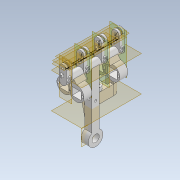
# Autodesk Inventor part: base_hand
Saved by Autodesk Inventor 2020.2 (Build 242310000, 310)
## iProperties
Created: 2020-04-08
Part Number: base_hand
Material: Generic
Document SubType Name: Modeling
Designer: Bardo91
Density: 1 g/cm^3
Appearance: Default
Author: Bardo91
Autodesk Inventor part; units mm, degrees
ref_plane "YZ Plane" through (0, 0, 0) normal (1, 0, 0) x (0, 1, 0)
sketch "Sketch1" plane through (0, 0, 0) normal (1, 0, 0) x (0, 1, 0)
  line L0 (0, 0) -> (0, -24)
  line L1 (0, -24) -> (0, -48)
  line L2 (0, -48) -> (0, -72)
  line L3 (0, -24) -> (5, -24)
  line L4 (0, -48) -> (8, -48)
  line L5 (0, -72) -> (5, -72)
  dimension "d0" = 24
  dimension "d1" = 24
  dimension "d2" = 24
  dimension "d4" = 5
  dimension "d5" = 8
  dimension "d6" = 5
  constraints: 12 end point, 2 horizontal, 2 point on line, 1 perpendicular, 1 vertical
  measures "d0" distance of L0.start L0.end
  measures "d1" distance of L0.end L1.end
  measures "d2" distance of L1.end L2.end
  measures "d4" distance of L0.end L3.end
  measures "d5" distance of L1.end L4.end
  measures "d6" distance of L2.end L5.end
ref_plane "Work Plane1" through (0, 5, -24) normal (0, 0, 1) x (1, 0, 0)
ref_plane "Work Plane3" through (0, 5, -72) normal (0, 0, 1) x (1, 0, 0)
ref_plane "Work Plane2" through (0, 8, -48) normal (0, 0, 1) x (1, 0, 0)
ref_plane "Work Plane4" through (0, 0, 0) normal (0, 0, 1) x (1, 0, 0)
sketch "Sketch2" plane through (0, 0, 0) normal (0, 0, 1) x (1, 0, 0)
  circle A0 centre (0, 0) radius 1.5
  circle A1 centre (0, 0) radius 5
  line L0 (0, 0) -> (0, -15)
  circle A2 centre (0, -15) radius 5
  line L1 (5, -15) -> (5, 0)
  line L2 (-5, -15) -> (-5, 0)
  dimension "d7" = 3
  dimension "d8" = 10
  dimension "d80" = 15
  dimension "d81" = 10
  constraints: 6 end point, 4 point on circle, 3 centre point, 3 coincident, 2 tangent, 2 vertical, 1 parallel
  measures "d7" diameter of A0
  measures "d8" diameter of A1
  measures "d80" distance of L0.start L0.end
  measures "d81" diameter of A2
extrude "pinky_joint" add sketch "Sketch2" along normal mid plane 8
sketch "Sketch18" plane through (0, 0, 4) normal (0, 0, 1) x (1, 0, 0)
  line L0 (0, 0) -> (0, -6)
  line L1 (0, -6) -> (0, -9)
  line L2 (0, 0) -> (1.058, -6)
  line L3 (0, 0) -> (6.0926, 0) construction
  line L4 (1.058, -6) -> (0, -6)
  line L5 (1.058, -6) -> (1.5869, -9)
  line L6 (1.5869, -9) -> (0, -9)
  dimension "d82" = 6
  dimension "d83" = 3
  dimension "d84" = 80
  constraints: 14 end point, 2 horizontal, 2 point on line, 1 equal length, 1 parallel, 1 vertical
  measures "d82" distance of L0.start L0.end
  measures "d83" distance of L0.end L1.end
  measures "d84" angle of L2 L3
extrude "lock" add sketch "Sketch18" along normal blind 3 contours L4 L5 L6 L1
ref_plane "Work Plane5" through (0, 0, 0) normal (0, 0, 1) x (1, 0, 0)
mirror "Mirror1" about plane through (0, 0, 0) normal (0, 0, 1) of "lock"
chamfer "Chamfer1" distance 3 angle 45 2 edges at (0, -7.5, 4) (0, -7.5, -4)
ref_plane "Work Plane6" through (0, 5, 0) normal (0, 1, 0) x (-1, 0, 0)
sketch "Sketch19" plane through (0, 5, 0) normal (0, 1, 0) x (-1, 0, 0)
  line L0 (0, 0) -> (-3, 0)
  circle A0 centre (-3, 0) radius 1.25
  dimension "d90" = 3
  dimension "thread_hole" = 2.5
  constraints: 2 end point, 1 centre point, 1 coincident, 1 horizontal
  measures "d90" distance of L0.start L0.end
  measures "thread_hole" diameter of A0
extrude "thread_hole" cut sketch "Sketch19" against normal through all
sketch "Sketch20" plane through (0, 0, 0) normal (0, 1, 0) x (-1, 0, 0)
  line L0 (0, 0) -> (-3, 0)
  circle A0 centre (-3, 0) radius 1.25
  line L1 (-3, -1.25) -> (-5, -1.25)
  line L2 (-5, -4) -> (-5, 4) projected
  line L3 (-3, 1.25) -> (-5, 1.25)
  line L4 (0, 0) -> (0, 2.405)
  dimension "d94" = 3
  dimension "d95" = 2.5
  constraints: 8 end point, 2 horizontal, 2 point on circle, 2 point on line, 1 centre point, 1 coincident, 1 parallel, 1 vertical
  measures "d94" distance of L0.start L0.end
  measures "d95" diameter of A0
revolve "Revolution2" cut sketch "Sketch20" angle 180 about axis through (0, 0, 0) along (0, 0, 1)
sketch "Sketch22" plane through (5, -15, 4) normal (1, 0, 0) x (0, 0, -1)
  line L0 (8, 0) -> (0, 0) projected
  line L1 (4, 0) -> (4, 1)
  circle A0 centre (4, 1) radius 1
  line L2 (4, 1) -> (4, 5)
  circle A1 centre (4, 5) radius 1
  point P0 (4, 15)
  dimension "d100" = 1
  dimension "d101" = 2
  dimension "d104" = 4
  dimension "d105" = 2
  constraints: 4 end point, 2 centre point, 2 coincident, 2 vertical, 1 midpoint
  measures "d100" distance of L1.start L1.end
  measures "d101" diameter of A0
  measures "d104" distance of L2.start L2.end
  measures "d105" diameter of A1
extrude "pinky_flector_holder" cut sketch "Sketch22" against normal up to surface round surface about axis through (3, 5, 0) along (0, -1, 0) radius 1.25 far side no
sketch "Sketch23" plane through (0, 0, -4) normal (0, 0, -1) x (-1, 0, 0)
  arc A0 (-5, -15) -> (5, -15) centre (0, -15) ccw projected
  circle A1 centre (0, -15) radius 5
  point P0 (0, 0)
  constraints: 1 coincident, 3 other
extrude "finger_union" add sketch "Sketch23" along normal blind 72
sketch "Sketch24" plane through (-5, 0, -1.25) normal (0, 1, 0) x (1, 0, 0)
  arc A0 (2, -2.5) -> (2, 0) centre (2, -1.25) ccw projected
  circle A1 centre (2, -1.25) radius 1.25
  point P0 (5, -1.25)
  constraints: 1 coincident, 3 other
extrude "pinky_actuator_hole" cut sketch "Sketch24" against normal through all
ref_plane "Work Plane7" through (0, 5, -24) normal (0, 0, -1) x (-1, 0, 0)
sketch "Sketch25" plane through (0, 5, -24) normal (0, 0, -1) x (-1, 0, 0)
  arc A0 (5, -5) -> (-5, -5) centre (0, -5) ccw projected
  circle A1 centre (0, 0) radius 1.5
  circle A2 centre (0, 0) radius 5
  line L0 (5, -5) -> (5, -20) projected
  line L1 (5, 0) -> (5, -20)
  line L2 (-5, -20) -> (-5, -5) projected
  line L3 (-5, 0) -> (-5, -20)
  circle A3 centre (0, -20) radius 5 projected
  circle A4 centre (0, -20) radius 5
  point P0 (-5, -5)
  point P1 (5, -5)
  dimension "d112" = 3
  dimension "d113" = 10
  constraints: 4 end point, 3 point on circle, 2 centre point, 2 coincident, 2 collinear, 1 horizontal alignment, 2 other
  measures "d112" diameter of A1
  measures "d113" diameter of A2
extrude "ring_base" add sketch "Sketch25" along normal mid plane 8 contours L0 A3 L2 A0 A2 | A0 A2 L1 | A2 A0 A1 | A0 A1 A2 | A0 L3 A2
sketch "Sketch26" plane through (0, 5, -20) normal (0, 0, 1) x (1, 0, 0)
  line L0 (0, 0) -> (0, -6)
  line L1 (0, -6) -> (0, -9)
  line L2 (0, 0) -> (1.5869, -9)
  line L3 (0, 0) -> (9.1388, 0) construction
  line L4 (1.5869, -9) -> (0, -9)
  line L5 (0, -6) -> (1.058, -6)
  point P0 (0, -5)
  dimension "d116" = 6
  dimension "d117" = 3
  dimension "d118" = 80
  constraints: 12 end point, 2 horizontal, 2 vertical, 1 equal length, 1 parallel, 1 point on line
  measures "d116" distance of L0.start L0.end
  measures "d117" distance of L0.end L1.end
  measures "d118" angle of L2 L3
extrude "ring_lock" add sketch "Sketch26" along normal blind 3 contours L5 L2 L4 L1
mirror "Mirror2" about plane through (0, 5, -24) normal (0, 0, -1) of "ring_lock"
chamfer "Chamfer2" distance 3 angle 45 2 edges at (0, -2.5, -20) (0, -2.5, -28)
ref_plane "Work Plane8" through (0, 8, -48) normal (0, 0, -1) x (-1, 0, 0)
ref_plane "Work Plane9" through (0, 5, -72) normal (0, 0, -1) x (-1, 0, 0)
sketch "Sketch27" plane through (0, 8, -48) normal (0, 0, -1) x (-1, 0, 0)
  circle A0 centre (0, 0) radius 1.5
  circle A1 centre (0, 0) radius 5
  line L0 (5, -8) -> (5, -23) projected
  line L1 (5, 0) -> (5, -23)
  arc A2 (5, -23) -> (-5, -23) centre (0, -23) ccw projected
  line L2 (-5, 0) -> (-5, -23)
  point P0 (0, -8)
  point P1 (5, -8)
  dimension "d124" = 3
  dimension "d125" = 10
  constraints: 4 end point, 2 centre point, 2 point on circle, 2 vertical, 1 coincident, 1 tangent
  measures "d124" diameter of A0
  measures "d125" diameter of A1
extrude "middle_base" add sketch "Sketch27" along normal mid plane 8
ref_plane "Work Plane11" through (5, 8, -44) normal (0, 1, 0) x (-1, 0, 0)
ref_plane "Work Plane10" through (5, 5, -20) normal (0, 1, 0) x (-1, 0, 0)
sketch "Sketch28" plane through (0, 5, -72) normal (0, 0, -1) x (-1, 0, 0)
  circle A0 centre (0, 0) radius 1.5
  circle A1 centre (0, 0) radius 5
  line L0 (5, 3) -> (5, -20) projected
  line L1 (5, 0) -> (5, -20)
  line L2 (-5, -20) -> (-5, 3) projected
  line L3 (-5, 0) -> (-5, -20)
  arc A2 (5, -20) -> (-5, -20) centre (0, -20) ccw projected
  circle A3 centre (0, -20) radius 5
  point P0 (0, -5)
  dimension "d128" = 3
  dimension "d129" = 10
  constraints: 4 end point, 2 centre point, 2 coincident, 2 collinear, 2 point on circle, 2 point on line, 1 horizontal alignment, 1 tangent, 2 other
  measures "d128" diameter of A0
  measures "d129" diameter of A1
extrude "index_base" add sketch "Sketch28" along normal mid plane 8 contours A1 | L0 A2 L2 A1
sketch "Sketch39" plane through (5, 5, -20) normal (0, 1, 0) x (-1, 0, 0)
  line L0 (10, -8) -> (10, 0) projected
  line L1 (10, -4) -> (0, -4)
  line L2 (0, -8) -> (0, 0) projected
  line L3 (5, -4) -> (1.5, -4)
  circle A0 centre (1.5, -4) radius 1.25
  line L4 (1.5, -5.25) -> (0, -5.25)
  line L5 (1.5, -2.75) -> (0, -2.75)
  line L6 (5, -4) -> (5, -5.6429)
  line L7 (0, -5.25) -> (0, -2.75)
  point P0 (5, 20)
  dimension "d165" = 3.5
  dimension "d166" = 2.5
  constraints: 12 end point, 3 midpoint, 3 point on line, 2 perpendicular, 2 point on circle, 1 centre point, 1 coincident, 1 collinear, 1 tangent, 1 vertical
  measures "d165" distance of L3.start L3.end
  measures "d166" diameter of A0
revolve "ring_1" cut sketch "Sketch39" angle 180 about axis through (0, 5, -24) along (0, 0, 1)
sketch "Sketch40" plane through (3.5, 5, -22.75) normal (0, 1, 0) x (1, 0, 0)
  arc A0 (0, 2.5) -> (0, 0) centre (0, 1.25) ccw projected
  circle A1 centre (0, 1.25) radius 1.25
  point P0 (-3.5, -22.75)
  constraints: 1 coincident, 3 other
extrude "ring_2" cut sketch "Sketch40" against normal through all
sketch "Sketch41" plane through (5, -15, -28) normal (1, 0, 0) x (0, 0, -1)
  line L0 (0, 0) -> (-8, 0) projected
  line L1 (-4, 0) -> (-4, 1)
  line L2 (-4, 1) -> (-4, 5)
  circle A0 centre (-4, 5) radius 1
  circle A1 centre (-4, 1) radius 1
  point P0 (-28, 15)
  dimension "d170" = 1
  dimension "d171" = 4
  dimension "d172" = 2
  dimension "d173" = 2
  constraints: 4 end point, 2 centre point, 2 coincident, 1 midpoint, 1 point on line, 1 vertical
  measures "d170" distance of L1.start L1.end
  measures "d171" distance of L1.end L2.end
  measures "d172" diameter of A0
  measures "d173" diameter of A1
extrude "ring_3" cut sketch "Sketch41" against normal up to surface round surface about axis through (3.5, 5, -24) along (0, -1, 0) radius 1.25 far side no
sketch "Sketch42" plane through (-5, 5, -22.75) normal (0, 1, 0) x (1, 0, 0)
  arc A0 (1.5, 0) -> (1.5, 2.5) centre (1.5, 1.25) ccw projected
  circle A1 centre (1.5, 1.25) radius 1.25
  point P0 (5, -22.75)
  constraints: 1 coincident, 3 other
extrude "ring_4" cut sketch "Sketch42" against normal through all
sketch "Sketch30" plane through (5, 8, -44) normal (0, 1, 0) x (-1, 0, 0)
  line L0 (10, -8) -> (10, 0) projected
  line L1 (10, -4) -> (0, -4)
  line L2 (0, 0) -> (0, -8) projected
  line L3 (5, -4) -> (1.5, -4)
  circle A0 centre (1.5, -4) radius 1.25
  line L4 (1.5, -5.25) -> (0, -5.25)
  line L5 (1.5, -2.75) -> (0, -2.75)
  line L6 (5, -4) -> (5, -4.8662)
  point P0 (5, 44)
  dimension "d135" = 3.5
  dimension "d136" = 2.5
  constraints: 10 end point, 3 midpoint, 3 point on line, 2 point on circle, 1 centre point, 1 coincident, 1 parallel, 1 perpendicular, 1 tangent, 1 vertical
  measures "d135" distance of L3.start L3.end
  measures "d136" diameter of A0
revolve "middle_1" cut sketch "Sketch30" angle 180 about axis through (0, 8, -48) along (0, 0, 1)
sketch "Sketch34" plane through (3.5, 8, -49.25) normal (0, 1, 0) x (1, 0, 0)
  arc A0 (0, 0) -> (0, -2.5) centre (0, -1.25) ccw projected
  circle A1 centre (0, -1.25) radius 1.25
  point P0 (-3.5, -49.25)
  point P1 (0, -2.5)
  constraints: 1 coincident, 3 other
extrude "middle_2" cut sketch "Sketch34" against normal through all
sketch "Sketch35" plane through (5, -15, -52) normal (1, 0, 0) x (0, 0, -1)
  line L0 (0, 0) -> (-8, 0) projected
  line L1 (-4, 0) -> (-4, 1)
  line L2 (-4, 1) -> (-4, 5)
  circle A0 centre (-4, 1) radius 1
  circle A1 centre (-4, 5) radius 1
  point P0 (-52, 15)
  dimension "d151" = 1
  dimension "d152" = 4
  dimension "d153" = 2
  dimension "d154" = 2
  constraints: 4 end point, 2 centre point, 2 coincident, 1 midpoint, 1 point on line, 1 vertical
  measures "d151" distance of L1.start L1.end
  measures "d152" distance of L1.end L2.end
  measures "d153" diameter of A0
  measures "d154" diameter of A1
extrude "middle_3" cut sketch "Sketch35" against normal up to surface round surface about axis through (3.5, 8, -48) along (0, -1, 0) radius 1.25 far side no
sketch "Sketch43" plane through (-5, 8, -49.25) normal (0, 1, 0) x (1, 0, 0)
  arc A0 (1.5, -2.5) -> (1.5, 0) centre (1.5, -1.25) ccw projected
  circle A1 centre (1.5, -1.25) radius 1.25
  point P0 (5, -49.25)
  point P1 (1.5, 0)
  constraints: 1 centre point, 1 coincident
extrude "middle_4" cut sketch "Sketch43" against normal through all
sketch "Sketch31" plane through (5, 5, -20) normal (0, 1, 0) x (-1, 0, 0)
  line L0 (10, -48) -> (10, -56) projected
  line L1 (10, -52) -> (0, -52)
  line L2 (0, -56) -> (0, -48) projected
  line L3 (5, -52) -> (1.5, -52)
  circle A0 centre (1.5, -52) radius 1.25
  line L4 (1.5, -53.25) -> (0, -53.25)
  line L5 (1.5, -50.75) -> (0, -50.75)
  line L6 (5, -52) -> (5, -50.2742)
  point P0 (5, 20)
  dimension "d138" = 3.5
  dimension "d139" = 2.5
  constraints: 10 end point, 3 midpoint, 3 point on line, 2 perpendicular, 2 point on circle, 1 centre point, 1 coincident, 1 tangent, 1 vertical
  measures "d138" distance of L3.start L3.end
  measures "d139" diameter of A0
revolve "index_1" cut sketch "Sketch31" angle 180 about axis through (0, 5, -72) along (0, 0, 1)
sketch "Sketch36" plane through (3.5, 5, -70.75) normal (0, 1, 0) x (1, 0, 0)
  arc A0 (0, 2.5) -> (0, 0) centre (0, 1.25) ccw projected
  circle A1 centre (0, 1.25) radius 1.25
  point P0 (-3.5, -70.75)
  constraints: 1 coincident, 3 other
extrude "index_2" cut sketch "Sketch36" against normal through all
sketch "Sketch37" plane through (5, -15, -76) normal (1, 0, 0) x (0, 0, -1)
  line L0 (-4, 0) -> (-4, 1)
  line L1 (-4, 1) -> (-4, 5)
  circle A0 centre (-4, 5) radius 1
  circle A1 centre (-4, 1) radius 1
  line L2 (-8, 0) -> (-8, 20) projected
  line L3 (0, 0) -> (0, 20) projected
  point P0 (-76, 15)
  dimension "d159" = 1
  dimension "d160" = 4
  dimension "d161" = 2
  dimension "d162" = 2
  dimension "d434" = 4
  constraints: 4 end point, 2 centre point, 2 coincident, 1 point on line, 1 vertical
  measures "d159" distance of L0.start L0.end
  measures "d160" distance of L0.end L1.end
  measures "d161" diameter of A0
  measures "d162" diameter of A1
  measures "d434" distance between parallel lines of L3 L1
extrude "index_3" cut sketch "Sketch37" against normal up to surface round surface about axis through (3.5, 5, -72) along (0, -1, 0) radius 1.25 far side no
sketch "Sketch44" plane through (-5, 5, -70.75) normal (0, 1, 0) x (1, 0, 0)
  arc A0 (1.5, 0) -> (1.5, 2.5) centre (1.5, 1.25) ccw projected
  circle A1 centre (1.5, 1.25) radius 1.25
  point P0 (5, -70.75)
  point P1 (1.5, 0)
  constraints: 1 coincident, 3 other
extrude "index_4" cut sketch "Sketch44" against normal through all
sketch "Sketch46" plane through (0, 5, -20) normal (0, 0, 1) x (1, 0, 0)
  arc A0 (-5, -20) -> (5, -20) centre (0, -20) ccw projected
  circle A1 centre (9, -35) radius 10
  line L0 (9, -25) -> (5, -20)
  line L1 (-1, -35) -> (-5, -20)
  line L2 (9, -35) -> (15, -35)
  line L3 (15, -35) -> (15, -30)
  line L4 (15, -30) -> (3, -30)
  line L5 (3, -30) -> (3, -40)
  line L6 (3, -40) -> (15, -40)
  line L7 (15, -40) -> (15, -35)
  line L8 (15.2, -35) -> (15.2, -29.8)
  line L9 (15.2, -29.8) -> (2.8, -29.8)
  line L10 (2.8, -29.8) -> (2.8, -40.2)
  line L11 (2.8, -40.2) -> (15.2, -40.2)
  line L12 (15.2, -40.2) -> (15.2, -35)
  point P0 (0, -5)
  point P1 (18.9875, -34.5)
  point P2 (18.9875, -35.5)
  point P3 (-4.3361, -22.4896)
  dimension "d369" = 15
  dimension "d370" = 9
  dimension "d371" = 6
  dimension "d372" = 5
  dimension "d373" = 12
  dimension "d374" = 10
  dimension "d375" = 0.2
  constraints: 26 end point, 7 perpendicular, 5 point on circle, 2 collinear, 1 centre point, 1 horizontal, 1 point on line, 4 other
  measures "d369" vertical distance of A0.centre L2.start
  measures "d370" horizontal distance of A0.centre L2.start
  measures "d371" distance of L2.start L2.end
  measures "d372" distance of L2.end L3.end
  measures "d373" distance of L3.end L4.end
  measures "d374" distance of L4.end L5.end
  measures "d375" distance between parallel lines of L7 L12
sketch "Sketch51" plane through (0, 8, -52) normal (0, 0, -1) x (-1, 0, 0)
  arc A0 (-4.9962, -22.8052) -> (-4.9944, -22.7631) centre (0, -23) ccw
  line L0 (0, -23) -> (0, -38)
  line L1 (0, -38) -> (-9, -38)
  circle A1 centre (-9, -38) radius 10
  arc A2 (-5, -23) -> (5, -23) centre (0, -23) ccw projected
  line L2 (-9, -28) -> (-5, -23)
  line L3 (1, -38) -> (5, -23)
  line L4 (-9, -38) -> (-15, -38)
  line L5 (-15, -38) -> (-15, -33)
  line L6 (-15, -33) -> (-3, -33)
  line L7 (-3, -33) -> (-3, -43)
  line L8 (-3, -43) -> (-15, -43)
  line L9 (-15, -43) -> (-15, -38)
  line L10 (-2.8, -43.2) -> (-2.8, -32.8)
  line L11 (-2.8, -32.8) -> (-15.2, -32.8)
  line L12 (-15.2, -32.8) -> (-15.2, -38)
  line L13 (-15.2, -38) -> (-15.2, -43.2)
  line L14 (-15.2, -43.2) -> (-2.8, -43.2)
  point P0 (0, -5)
  point P1 (0, -5)
  point P2 (0.9875, -37.5)
  point P3 (-7.2605, -28.1524)
  point P4 (-5, -23)
  point P5 (5, -23)
  point P6 (4.3361, -25.4896)
  point P7 (-18.9875, -38.5)
  point P8 (-18.9875, -37.5)
  dimension "d227" = 15
  dimension "d230" = 20
  dimension "d235" = 5
  dimension "d237" = 9
  dimension "d382" = 6
  dimension "d383" = 5
  dimension "d384" = 12
  dimension "d385" = 10
  dimension "d386" = 0.2
  constraints: 30 end point, 10 perpendicular, 8 point on circle, 2 centre point, 2 coincident, 1 horizontal, 1 point on line, 1 vertical, 4 other
  measures "d227" distance of L0.start L0.end
  measures "d230" diameter of A1
  measures "d235" radius of A0
  measures "d237" distance of L0.end L1.end
  measures "d382" distance of L4.start L4.end
  measures "d383" distance of L4.end L5.end
  measures "d384" distance of L5.end L6.end
  measures "d385" distance of L6.end L7.end
  measures "d386" distance between parallel lines of L7 L10
extrude "ring_motor" add sketch "Sketch46" along normal blind 14 contours A0 L0 A1 L1 | A1
extrude "middle_motor" add sketch "Sketch51" along normal blind 14 contours A0 L0 A1 L2 | A0 L3 A1 L0 | A1
sketch "Sketch52" plane through (0, 5, -68) normal (0, 0, 1) x (1, 0, 0)
  arc A0 (-4.9995, -20.0687) -> (4.9995, -20.0687) centre (0, -20) ccw
  line L0 (0, -20) -> (0, -35)
  circle A1 centre (-9, -35) radius 10
  arc A2 (-4.3361, -22.4896) -> (5, -20) centre (0, -20) ccw projected
  line L1 (5, -20) -> (9, -25) projected
  line L2 (1, -35) -> (5, -20)
  line L3 (-4.3361, -22.4896) -> (-8.7782, -25.0025)
  line L4 (-9, -35) -> (-3, -35)
  line L5 (-3, -35) -> (-3, -40)
  line L6 (-3, -40) -> (-15, -40)
  line L7 (-15, -40) -> (-15, -30)
  line L8 (-15, -30) -> (-3, -30)
  line L9 (-3, -30) -> (-3, -35)
  line L10 (-2.8, -40.2) -> (-2.8, -35)
  line L11 (-2.8, -35) -> (-2.8, -29.8)
  line L12 (-2.8, -29.8) -> (-15.2, -29.8)
  line L13 (-15.2, -29.8) -> (-15.2, -40.2)
  line L14 (-15.2, -40.2) -> (-2.8, -40.2)
  point P0 (0, -5)
  point P1 (0, -5)
  point P2 (0.9875, -34.5)
  point P3 (0.9875, -35.5)
  point P4 (11.9791, -34.5)
  point P5 (11.9791, -35.5)
  point P6 (-4.9558, -20.6637)
  point P7 (4.3361, -22.4896)
  point P8 (-18.9875, -35.5)
  point P9 (-18.9875, -34.5)
  point P10 (-4.3361, -22.4896)
  dimension "d254" = 5
  dimension "d392" = 15
  dimension "d393" = 9
  dimension "d394" = 6
  dimension "d395" = 5
  dimension "d396" = 12
  dimension "d397" = 10
  dimension "d398" = 0.2
  constraints: 28 end point, 9 perpendicular, 9 point on circle, 2 centre point, 2 coincident, 1 horizontal, 1 point on line, 1 vertical, 4 other
  measures "d254" radius of A0
  measures "d392" vertical distance of L4.start L0.start
  measures "d393" horizontal distance of L4.start L0.start
  measures "d394" distance of L4.start L4.end
  measures "d395" distance of L4.end L5.end
  measures "d396" distance of L5.end L6.end
  measures "d397" distance of L6.end L7.end
  measures "d398" distance between parallel lines of L5 L10
extrude "index_motor" add sketch "Sketch52" along normal blind 14 contours A0 L0 A1 L3 | A0 L2 A1 L0 | A1
sketch "Sketch53" plane through (0, 0, -4) normal (0, 0, -1) x (-1, 0, 0)
  arc A0 (-2, -15) -> (2, -15) centre (0, -15) ccw
  circle A1 centre (9, -30) radius 10
  line L0 (9, -20) -> (2, -15)
  line L1 (-1, -30) -> (-2, -15)
  arc A2 (-5, -15) -> (5, -15) centre (0, -15) ccw projected
  line L2 (15.2, -24.8) -> (2.8, -24.8) projected
  line L3 (15.2, -24.8) -> (2.8, -24.8)
  line L4 (2.8, -24.8) -> (2.8, -35.2) projected
  line L5 (2.8, -24.8) -> (2.8, -35.2)
  line L6 (2.8, -35.2) -> (15.2, -35.2) projected
  line L7 (2.8, -35.2) -> (15.2, -35.2)
  line L8 (15.2, -35.2) -> (15.2, -24.8)
  point P0 (0, 0)
  point P1 (11.9791, -34.5)
  point P2 (11.9791, -35.5)
  point P3 (-4.9558, -20.6637)
  point P4 (-0.0209, -34.5)
  point P5 (4.9558, -20.6637)
  point P6 (-4.9558, -20.6637)
  point P7 (-4.6607, -25.0901)
  point P8 (-0.0209, -35.5)
  point P9 (0, -5)
  point P10 (11.9791, -34.5)
  point P11 (11.9791, -35.5)
  point P12 (-4.9558, -20.6637)
  point P13 (-1.9823, -15.2655)
  dimension "d273" = 20
  dimension "d405" = 15
  dimension "d406" = 9
  constraints: 12 end point, 5 point on circle, 2 centre point, 2 coincident, 2 horizontal, 1 collinear, 1 perpendicular
  measures "d273" diameter of A1
  measures "d405" vertical distance of A0.centre A1.centre
  measures "d406" horizontal distance of A0.centre A1.centre
extrude "pinky_motor" add sketch "Sketch53" along normal blind 14
sketch "Sketch67" plane through (0, 8, -52) normal (0, 0, 1) x (1, 0, 0)
  circle A0 centre (9, -38) radius 10 projected
  circle A1 centre (9, -38) radius 10
  circle A2 centre (9, -38) radius 2.5
  point P0 (0, -8)
  constraints: 2 centre point, 2 coincident
extrude "Extrusion48" cut sketch "Sketch67" against normal blind 3
sketch "Sketch69" plane through (0, 5, -68) normal (0, 0, -1) x (-1, 0, 0)
  arc A0 (-1, -35) -> (8.7782, -25.0025) centre (9, -35) ccw projected
  circle A1 centre (9, -35) radius 10
  arc A2 (-2.8, -40.0557) -> (-2.8, -29.9443) centre (-9, -35) ccw projected
  circle A3 centre (9, -35) radius 2.5
  point P0 (0, -5)
  point P1 (8.7782, -25.0025)
  point P2 (0, -39.3589)
  point P3 (19, -35)
  dimension "d399" = 5
  constraints: 2 centre point, 2 coincident, 1 tangent
  measures "d399" diameter of A3
extrude "Extrusion50" cut sketch "Sketch69" against normal blind 3
sketch "Sketch65" plane through (0, 5, -20) normal (0, 0, -1) x (-1, 0, 0)
  arc A0 (-9, -25) -> (1, -35) centre (-9, -35) ccw projected
  circle A1 centre (-9, -35) radius 10
  circle A2 centre (-9, -35) radius 2.5
  point P0 (0, -5)
  point P1 (1, -35)
  dimension "d376" = 5
  constraints: 2 coincident, 1 centre point, 3 other
  measures "d376" diameter of A2
extrude "Extrusion46" cut sketch "Sketch65" against normal blind 3
sketch "Sketch71" plane through (0, 0, -4) normal (0, 0, 1) x (1, 0, 0)
  arc A0 (-9, -20) -> (1, -30) centre (-9, -30) ccw projected
  circle A1 centre (-9, -30) radius 10
  circle A2 centre (-9, -30) radius 2.5
  point P0 (0, 0)
  point P1 (-9, -20)
  point P2 (0, -34.3589)
  point P3 (0, -34.3589)
  dimension "d407" = 5
  constraints: 2 coincident, 1 centre point, 3 other
  measures "d407" diameter of A2
extrude "Extrusion52" cut sketch "Sketch71" against normal blind 3
sketch "Sketch73" plane through (0, 5, -17) normal (0, 0, -1) x (-1, 0, 0)
  line L0 (-15.2, -29.8) -> (-15.2, -40.2) projected
  line L1 (-15.2, -35) -> (-19, -35)
  arc A0 (-9, -25) -> (0, -39.3589) centre (-9, -35) ccw projected
  line L2 (-2.8, -40.2) -> (-2.8, -29.8) projected
  line L3 (-2.8, -35) -> (1, -35)
  arc A1 (0, -39.3589) -> (-9, -25) centre (-9, -35) ccw projected
  circle A2 centre (-0.9, -35) radius 1.5
  circle A3 centre (-17.1, -35) radius 1.5
  point P0 (0, -5)
  dimension "d412" = 3
  dimension "d413" = 3
  constraints: 4 end point, 4 midpoint, 2 centre point, 2 horizontal, 2 point on circle
  measures "d412" diameter of A2
  measures "d413" diameter of A3
extrude "Extrusion54" cut sketch "Sketch73" against normal through all both and the other way through all contours A3 L1 | L1 A3
sketch "Sketch74" plane through (0, 5, -20) normal (0, 0, -1) x (-1, 0, 0)
  line L0 (15.2, -40.2) -> (15.2, -29.8) projected
  line L1 (15.2, -35) -> (19, -35)
  arc A0 (0, -39.3589) -> (8.7782, -25.0025) centre (9, -35) ccw projected
  circle A1 centre (17.1, -35) radius 1.5
  point P0 (0, -5)
  dimension "d416" = 3
  constraints: 2 end point, 2 midpoint, 1 centre point, 1 horizontal, 1 point on circle
  measures "d416" diameter of A1
extrude "Extrusion55" cut sketch "Sketch74" against normal through all both and the other way through all
sketch "Sketch54" plane through (0, 8, -44) normal (0, 0, 1) x (1, 0, 0)
  line L0 (0, 0) -> (0, -6)
  line L1 (0, -6) -> (0, -9)
  circle A0 centre (0, 0) radius 1.5 projected
  line L2 (0, 0) -> (1.5869, -9)
  line L3 (0, 0) -> (9.1388, 0) construction
  line L4 (1.5869, -9) -> (0, -9)
  line L5 (-2.25, -3) -> (-2.25, -27.4651) projected
  line L6 (0, -6) -> (1.058, -6)
  point P0 (0, -8)
  dimension "d282" = 6
  dimension "d283" = 3
  dimension "d284" = 80
  constraints: 12 end point, 2 point on line, 1 equal length, 1 horizontal, 1 parallel, 1 perpendicular, 1 vertical
  measures "d282" distance of L0.start L0.end
  measures "d283" distance of L0.end L1.end
  measures "d284" angle of L2 L3
extrude "lock_middle" add sketch "Sketch54" along normal blind 3 contours L6 L2 L4 L1
mirror "Mirror3" about plane through (0, 8, -48) normal (0, 0, -1) of "lock_middle"
chamfer "Chamfer3" distance 3 angle 45 2 edges at (0, 0.5, -44) (0, 0.5, -52)
sketch "Sketch55" plane through (0, 5, -68) normal (0, 0, 1) x (1, 0, 0)
  line L0 (0, 0) -> (0, -6)
  line L1 (0, 0) -> (6, 0) construction
  line L2 (0, -6) -> (0, -9)
  line L3 (0, 0) -> (1.5869, -9)
  line L4 (0, 0) -> (9.1388, 0) construction
  line L5 (1.5869, -9) -> (0, -9)
  line L6 (-2.25, 0) -> (-2.25, -24.4651) projected
  line L7 (0, -6) -> (1.058, -6)
  point P0 (0, -5)
  dimension "d290" = 6
  dimension "d291" = 90
  dimension "d292" = 3
  dimension "d293" = 80
  constraints: 14 end point, 2 equal length, 2 horizontal, 2 point on line, 1 parallel, 1 perpendicular, 1 vertical
  measures "d290" distance of L0.start L0.end
  measures "d291" angle of L0 L1
  measures "d292" distance of L0.end L2.end
  measures "d293" angle of L3 L4
extrude "lock_index" add sketch "Sketch55" along normal blind 3 contours L7 L3 L5 L2
mirror "Mirror4" about plane through (0, 5, -72) normal (0, 0, -1) of "lock_index"
chamfer "Chamfer4" distance 3 angle 45 2 edges at (0, -2.5, -76) (0, -2.5, -68)
sketch "Sketch56" plane through (5, -15, 4) normal (1, 0, 0) x (0, 0, -1)
  circle A0 centre (4, 5) radius 1 projected
  circle A1 centre (4, 5) radius 1
  circle A2 centre (4, 5) radius 2
  circle A3 centre (4, 1) radius 1 projected
  circle A4 centre (4, 1) radius 1
  circle A5 centre (4, 1) radius 2
  circle A6 centre (28, 5) radius 1 projected
  circle A7 centre (28, 5) radius 1
  circle A8 centre (28, 5) radius 2
  circle A9 centre (28, 1) radius 1 projected
  circle A10 centre (28, 1) radius 1
  circle A11 centre (28, 1) radius 2
  circle A12 centre (52, 5) radius 1 projected
  circle A13 centre (52, 5) radius 1
  circle A14 centre (52, 5) radius 2
  circle A15 centre (52, 1) radius 1 projected
  circle A16 centre (52, 1) radius 1
  circle A17 centre (52, 1) radius 2
  circle A18 centre (76, 5) radius 1 projected
  circle A19 centre (76, 5) radius 1
  circle A20 centre (76, 5) radius 2
  circle A21 centre (76, 1) radius 1 projected
  circle A22 centre (76, 1) radius 1
  circle A23 centre (76, 1) radius 2
  point P0 (4, 15)
  point P1 (4, 0)
  point P2 (28, 0)
  point P3 (52, 0)
  point P4 (76, 0)
  dimension "d299" = 4
  dimension "d300" = 4
  dimension "d301" = 4
  dimension "d302" = 4
  dimension "d303" = 4
  dimension "d304" = 4
  dimension "d305" = 4
  dimension "d306" = 4
  constraints: 16 centre point, 16 coincident, 4 vertical alignment
  measures "d299" diameter of A2
  measures "d300" diameter of A5
  measures "d301" diameter of A8
  measures "d302" diameter of A11
  measures "d303" diameter of A14
  measures "d304" diameter of A17
  measures "d305" diameter of A20
  measures "d306" diameter of A23
extrude "reinforcement_thread_screw" add sketch "Sketch56" along normal blind 2
ref_plane "Work Plane12" through (-5, -15, -76) normal (0, 1, 0) x (-1, 0, 0)
sketch "Sketch57" plane through (-5, -15, -76) normal (0, 1, 0) x (-1, 0, 0)
  line L0 (-10, 0) -> (-10, 80) projected
  line L1 (-10, 40) -> (0, 40)
  line L2 (0, 0) -> (0, 80) projected
  line L3 (0, 40) -> (-4.5, 40)
  line L4 (0, 0) -> (0, 80) projected
  line L5 (-10, 45) -> (0, 45)
  line L6 (0, 45) -> (0, 35)
  line L7 (0, 35) -> (-10, 35)
  line L8 (-10, 35) -> (-10, 45)
  point P0 (-5, 76)
  point P1 (0, 45)
  dimension "d436" = 10
  dimension "d437" = 10
  dimension "d438" = 5
  constraints: 12 end point, 2 midpoint, 2 parallel, 2 point on line, 1 collinear, 1 horizontal, 1 perpendicular
  measures "d436" distance of L1.start L1.end
  measures "d437" distance between parallel lines of L7 L5
  measures "d438" distance between parallel lines of L7 L1
extrude "spine_hand" add sketch "Sketch57" against normal blind 80
ref_plane "Work Plane13" through (-5, -63, -76) normal (0, 1, 0) x (-1, 0, 0)
sketch "Sketch58" plane through (-5, -63, -76) normal (0, 1, 0) x (-1, 0, 0)
  circle A0 centre (15, 0) radius 10
  circle A1 centre (15, 20) radius 10
  line L0 (-0.5, 22) -> (4.5, 22) construction
  line L1 (21.2, 25.2) -> (8.8, 25.2)
  line L2 (8.8, 25.2) -> (8.8, 14.8)
  line L3 (8.8, 14.8) -> (21.2, 14.8)
  line L4 (21.2, 14.8) -> (21.2, 25.2)
  line L5 (21.2, 5.2) -> (8.8, 5.2)
  line L6 (8.8, 5.2) -> (8.8, -5.2)
  line L7 (8.8, -5.2) -> (21.2, -5.2)
  line L8 (21.2, -5.2) -> (21.2, 5.2)
  line L9 (15, 0) -> (15, 20)
  line L10 (-10, 35) -> (-10, 45) projected
  line L11 (-10, 40) -> (0, 40)
  line L12 (0, 45) -> (0, 35) projected
  line L13 (25, 0) -> (25, 20)
  line L14 (5, 0) -> (5, 20)
  line L15 (-10, 35) -> (5, 20)
  line L16 (0, 45) -> (21.29, 27.774)
  point P0 (-5, 76)
  point P1 (-1.1144, 14.5)
  point P2 (15, 10)
  point P3 (-5, 40)
  dimension "d442" = 20
  dimension "d443" = 20
  dimension "d444" = 5.2
  dimension "d445" = 6.2
  dimension "d446" = 5.2
  dimension "d447" = 6.2
  dimension "d448" = 12.4
  dimension "d449" = 10.4
  dimension "d450" = 12.4
  dimension "d451" = 10.4
  dimension "d452" = 20
  dimension "d453" = 20
  constraints: 30 end point, 6 perpendicular, 5 point on circle, 3 midpoint, 2 centre point, 2 tangent, 1 horizontal, 1 parallel, 1 vertical
  measures "d442" diameter of A1
  measures "d443" distance of L9.end L9.start
  measures "d444" distance from line of L9.end L1
  measures "d445" distance from line of L9.end L4
  measures "d446" distance from line of L7 L9.start
  measures "d447" distance from line of L9.start L6
  measures "d448" distance of L7.start L8.start
  measures "d449" distance of L5.end L7.start
  measures "d450" distance of L2.end L3.end
  measures "d451" distance of L3.end L1.start
  measures "d452" horizontal distance of point (-5, 40) L9.end
  measures "d453" horizontal distance of L9.end point (-5, 40)
extrude "thumb_motor_" add sketch "Sketch58" against normal blind 14
sketch "Sketch75" plane through (-5, -63, -76) normal (0, 1, 0) x (1, 0, 0)
  line L0 (-8.8, 5.2) -> (-8.8, -5.2) projected
  line L1 (-8.8, 0) -> (-6.9, 0)
  circle A0 centre (-6.9, 0) radius 1.5
  line L2 (-8.8, -14.8) -> (-8.8, -25.2) projected
  line L3 (-8.8, -20) -> (-6.9, -20)
  circle A1 centre (-6.9, -20) radius 1.5
  point P0 (5, -76)
  dimension "d428" = 1.9
  dimension "d429" = 3
  dimension "d430" = 1.9
  dimension "d431" = 3
  constraints: 4 end point, 2 centre point, 2 coincident, 2 horizontal, 2 midpoint
  measures "d428" distance of L1.start L1.end
  measures "d429" diameter of A0
  measures "d430" distance of L3.start L3.end
  measures "d431" diameter of A1
extrude "Extrusion56" cut sketch "Sketch75" against normal through all
ref_plane "Work Plane15" through (-0.5, -95, -33) normal (1, 0, 0) x (0, 1, 0)
sketch "Sketch76" plane through (-5, -63, -76) normal (0, 1, 0) x (1, 0, 0)
  arc A0 (-25, -20) -> (-21.29, -27.774) centre (-15, -20) ccw projected
  circle A1 centre (-15, -20) radius 10
  line L0 (-21.2, -14.8) -> (-21.2, -25.2) projected
  line L1 (-8.8, -14.8) -> (-21.2, -14.8) projected
  line L2 (-21.2, -25.2) -> (-8.8, -25.2)
  line L3 (-8.8, -25.2) -> (-8.8, -14.8)
  line L4 (-8.8, -14.8) -> (-21.2, -14.8)
  line L5 (-21.2, -14.8) -> (-21.2, -25.2)
  circle A2 centre (-6.9, -20) radius 1.5 projected
  circle A3 centre (-6.9, -20) radius 1.5
  point P0 (5, -76)
  point P1 (-11.7315, -29.821)
  point P2 (-12.1144, -14.5)
  point P3 (4.5, -27)
  point P4 (-5, -20)
  point P5 (1.1144, -14.5)
  point P6 (-15, -10)
  point P7 (0, -35.3516)
  point P8 (2.1563, -20.5671)
  point P9 (3.682, -23.0389)
  point P10 (-16.8224, -32.0236)
  point P11 (-21.29, -27.774)
  point P12 (-25, -20)
  constraints: 8 end point, 2 coincident, 2 parallel, 1 centre point, 1 horizontal, 1 perpendicular, 4 other
extrude "Extrusion57" add sketch "Sketch76" along normal blind 5
sketch "Sketch62" plane through (5, -15, -31) normal (1, 0, 0) x (0, 0, -1)
  line L0 (0, 0) -> (0, -80) projected
  line L1 (0, -45.1001) -> (10, -45.1001)
  line L2 (10, 0) -> (10, -80) projected
  line L3 (5, -45.1001) -> (5, -40.6001)
  circle A0 centre (5, -40.6001) radius 1.5
  point P0 (-31, 15)
  point P1 (0, -67)
  point P2 (9, -67)
  point P3 (0, -75.202)
  point P4 (10, -79)
  dimension "d349" = 4.5
  dimension "d350" = 3
  constraints: 4 end point, 1 centre point, 1 coincident, 1 horizontal, 1 midpoint, 1 perpendicular, 1 point on line, 2 other
  measures "d349" distance of L3.start L3.end
  measures "d350" diameter of A0
extrude "Extrusion43" cut sketch "Sketch62" against normal through all
sketch "Sketch63" plane through (3.753, -77, -41) normal (0, 0, -1) x (-1, 0, 0)
  line L0 (-1.247, 62) -> (-1.247, -18) projected
  line L1 (8.383, 62) -> (8.383, -13.202) projected
  line L2 (3.253, 14) -> (3.253, 24)
  circle A0 centre (3.253, 24) radius 1.5
  line L3 (8.383, 62) -> (8.383, 14) projected
  line L4 (8.383, 14) -> (-1.247, 14)
  line L5 (-1.247, 14) -> (8.753, 14) projected
  point P0 (3.753, 77)
  point P1 (-0.617, -17)
  point P2 (8.383, -17)
  point P3 (0, 14)
  point P4 (4.1915, 14)
  point P5 (-0.247, -13.202)
  point P6 (8.753, -13.202)
  point P7 (-1.247, -18)
  point P8 (8.253, 14)
  dimension "d353" = 10
  dimension "d354" = 3
  dimension "d367" = 4.5
  dimension "d368" = 0
  constraints: 4 end point, 1 centre point, 1 coincident, 1 collinear, 1 point on line, 1 vertical, 3 other
  measures "d353" distance of L2.start L2.end
  measures "d354" diameter of A0
  measures "d368" distance from line of L4 L2.start
extrude "Extrusion44" cut sketch "Sketch63" against normal through all
sketch "Sketch64" plane through (3.753, -77, -41) normal (0, 0, -1) x (-1, 0, 0)
  circle A0 centre (3.253, 24) radius 1.5 projected
  circle A1 centre (3.253, 24) radius 3
  line L0 (3.253, 27) -> (1.521, 27)
  line L1 (0.6549, 25.5) -> (1.521, 27)
  line L2 (0.6549, 22.5) -> (-0.2111, 24)
  line L3 (0.6549, 25.5) -> (-0.2111, 24)
  line L4 (3.253, 21) -> (1.521, 21)
  line L5 (0.6549, 22.5) -> (1.521, 21)
  line L6 (5.8511, 22.5) -> (4.9851, 21)
  line L7 (3.253, 21) -> (4.9851, 21)
  line L8 (5.8511, 25.5) -> (6.7171, 24)
  line L9 (5.8511, 22.5) -> (6.7171, 24)
  line L10 (3.253, 27) -> (4.9851, 27)
  line L11 (5.8511, 25.5) -> (4.9851, 27)
  point P0 (3.753, 77)
  dimension "d357" = 6
  dimension "d358" = 120
  dimension "d361" = 360
  constraints: 24 end point, 2 point on circle, 2 tangent, 1 centre point, 1 coincident, 1 horizontal, 31 other
  measures "d357" diameter of A1
  measures "d358" angle of L0 L1
extrude "Extrusion45" cut sketch "Sketch64" against normal blind 2
sketch "Sketch77" plane through (-5, -95, -41) normal (-1, 0, 0) x (0, 0, 1)
  line L0 (10, 0) -> (0, 0) projected
  line L1 (5, 0) -> (5, -5)
  circle A0 centre (5, -5) radius 5
  circle A1 centre (5, -5) radius 10
  point P0 (41, 95)
  dimension "d454" = 5
  dimension "d455" = 10
  dimension "d456" = 20
  constraints: 2 centre point, 2 coincident, 2 end point, 1 midpoint, 1 vertical
  measures "d454" distance of L1.start L1.end
  measures "d455" diameter of A0
  measures "d456" diameter of A1
extrude "Extrusion58" add sketch "Sketch77" against normal up to surface (10 mm away)
sketch "Sketch78" plane through (0, -15, -41) normal (0, 0, -1) x (-1, 0, 0)
  circle A0 centre (9.1717, -15.0472) radius 7.5
  point P0 (0, 15)
  dimension "d459" = 15
  constraints: 1 centre point
  measures "d459" diameter of A0
extrude "Extrusion59" cut sketch "Sketch78" against normal up to surface (10 mm away)
equation "\"d95\" = thread_hole"
body "Solid1"
